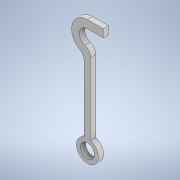
# Autodesk Inventor part: Hook
Saved by Autodesk Inventor 2022 (Build 260153000, 153)
## iProperties
Created: 2023-02-27
Part Number: Hook
Material: Generic
Document SubType Name: Modeling
Designer: zarek
Density: 1 g/cm^3
Appearance: Default
Author: zarek
Autodesk Inventor part; units mm, degrees
ref_plane "YZ Plane" through (0, 0, 0) normal (1, 0, 0) x (0, 1, 0)
ref_plane "XZ Plane" through (0, 0, 0) normal (0, 1, 0) x (-1, 0, 0)
ref_plane "XY Plane" through (0, 0, 0) normal (0, 0, 1) x (1, 0, 0)
sketch "Sketch1" plane through (0, 0, 0) normal (0, 0, 1) x (1, 0, 0)
  circle A0 centre (0, 0) radius 2.667
  circle A1 centre (0, 0) radius 4.167
  line L0 (-1.25, 3.9751) -> (1.25, 3.9751)
  line L1 (1.25, 3.9751) -> (1.25, 37.2251)
  line L2 (1.25, 37.2251) -> (-1.25, 37.2251)
  line L3 (-1.25, 37.2251) -> (-1.25, 3.9751)
  line L4 (0, 0) -> (0, 14.9208)
  circle A2 centre (0, 37.2251) radius 3
  circle A3 centre (0, 37.2251) radius 6
  line L5 (0, 43.2251) -> (6, 43.2251)
  line L6 (6, 43.2251) -> (6, 40.2251)
  line L7 (6, 40.2251) -> (0, 40.2251)
  point P0 (-1.25, 31.3567)
  point P1 (1.25, 3.9751)
  point P2 (1.25, 3.9751)
  point P3 (1.25, 34.4979)
  dimension "d1" = 8.334
  dimension "d5" = 6
  dimension "d6" = 12
  dimension "d0" = 5.334
  dimension "d2" = 1.25
  dimension "d3" = 1.25
  dimension "d4" = 33.25
  dimension "d7" = 6
  constraints: 16 end point, 4 horizontal, 3 coincident, 2 parallel, 2 perpendicular, 1 centre point, 1 midpoint, 1 vertical, 9 other
  measures "d0" diameter of A0
  measures "d2" distance between parallel lines of L3 L4
  measures "d3" distance between parallel lines of L1 L4
  measures "d4" distance between parallel lines of L0 L2
  measures "d7" distance from line of L6 L5.start
extrude "Extrusion1" add sketch "Sketch1" along normal blind 2 contours L0 A1 | L0 A1 L4 | L4 A1 L0 | L3 A3 L1 A1 | A3 L7 A2 L3 | L3 A2 L1 A3 | L5 L6 L7 A3
fillet "Fillet1" radius 3.175 2 edges at (1.25, 34.4979, 1) (-1.25, 31.3567, 1)
equation "\"d2\" = d3"
body "Solid1"
